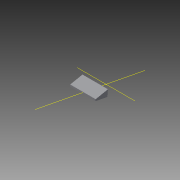
# Autodesk Inventor part: Prow
Saved by Autodesk Inventor 2015 (Build 190159000, 159)
## iProperties
Created: 2016-01-19
Part Number: Prow
Material: Generic
Document SubType Name: Modeling
Designer: sethbattis
Density: 1 g/cm^3
Appearance: Default
Author: sethbattis
Autodesk Inventor part; units mm, degrees
ref_plane "YZ Plane" through (0, 0, 0) normal (1, 0, 0) x (0, 1, 0)
ref_plane "XZ Plane" through (0, 0, 0) normal (0, 1, 0) x (-1, 0, 0)
ref_plane "XY Plane" through (0, 0, 0) normal (0, 0, 1) x (1, 0, 0)
sketch "Robot Front End" plane through (0, 0, 0) normal (1, 0, 0) x (0, 1, 0)
  circle A0 centre (127, -196.85) radius 127
  line L0 (304.8, 0) -> (177.8, 0)
  line L1 (177.8, 0) -> (177.8, 50.8)
  line L2 (209.55, 82.55) -> (273.05, 82.55)
  line L3 (304.8, 50.8) -> (304.8, 0)
  line L4 (0, -1177.7856) -> (0, 1643.8138) projected
  line L5 (-567.69, 0) -> (1050.29, 0) projected
  arc A1 (209.55, 82.55) -> (177.8, 50.8) centre (209.55, 50.8) ccw
  arc A2 (304.8, 50.8) -> (273.05, 82.55) centre (273.05, 50.8) ccw
  line L6 (241.3, 381) -> (0, 381) construction
  circle A3 centre (165.1, -196.85) radius 9.525
  circle A4 centre (241.3, -196.85) radius 25.4
  circle A5 centre (241.3, -196.85) radius 281.427 construction
  circle A6 centre (241.3, -196.85) radius 577.85 construction
  line L7 (165.1, -196.85) -> (241.3, -196.85) construction
  point P0 (0, 0)
  point P1 (177.8, 82.55)
  point P2 (304.8, 82.55)
  dimension "d76" = 254
  dimension "d77" = 127
  dimension "d78" = 82.55
  dimension "d79" = 304.8
  dimension "d80" = 196.85
  dimension "d81" = 31.75
  dimension "d82" = 381
  dimension "d104" = 19.05
  dimension "d105" = 165.1
  dimension "d110" = 50.8
  dimension "d128" = 76.2
  constraints: 12 end point, 6 centre point, 6 tangent, 5 point on line, 4 point on circle, 3 horizontal, 2 coincident, 2 parallel, 2 perpendicular, 1 collinear, 1 equal radius, 1 vertical alignment, 2 other
  measures "d76" diameter of A0
  measures "d77" distance of point (177.8, 82.55) point (304.8, 82.55)
  measures "d78" distance of L0.end point (177.8, 82.55)
  measures "d79" distance between parallel lines of L3 L4
  measures "d80" distance from line of A0.centre L5
  measures "d81" radius of A1
  measures "d82" distance between parallel lines of L5 L6
  measures "d104" diameter of A3
  measures "d105" distance from line of L4 L7.start
  measures "d110" diameter of A4
  measures "d128" distance of L7.start L7.end
sketch "Portcullis" plane through (0, 0, 0) normal (1, 0, 0) x (0, 1, 0)
  line L0 (0, 1071.5852) -> (76.2, 776.4639)
  line L1 (76.2, 776.4639) -> (76.2, 166.8639)
  line L2 (76.2, 166.8639) -> (0, -128.2574)
  line L3 (0, -1177.7856) -> (0, 1643.8138) projected
  line L4 (-567.69, 0) -> (1050.29, 0) projected
  line L5 (76.2, 379.7426) -> (285.0269, 379.7426) construction
  line L6 (203.2, 379.7426) -> (203.2, 475.769)
  line L7 (241.3, 381) -> (0, 381) projected
  circle A0 centre (241.3, -196.85) radius 577.85 construction
  point P0 (0, 0)
  dimension "d83" = 304.8
  dimension "d84" = 609.6
  dimension "d85" = 76.2
  dimension "d86" = 508
  dimension "d87" = 127
  constraints: 10 end point, 4 point on line, 2 vertical, 1 equal length, 1 horizontal, 1 point on circle
  measures "d83" distance of L0.start L0.end
  measures "d84" distance of L0.end L1.end
  measures "d85" distance between parallel lines of L3 L1
  measures "d86" distance from line of L2.end L5
  measures "d87" distance between parallel lines of L1 L6
sketch "Ball Attack" plane through (0, 0, 0) normal (1, 0, 0) x (0, 1, 0)
  line L0 (0, -1177.7856) -> (0, 1643.8138) construction
  circle A0 centre (241.3, -196.85) radius 281.427 construction
  circle A1 centre (241.3, -196.85) radius 577.85 construction
  circle A2 centre (241.3, -196.85) radius 25.4 construction
  circle A3 centre (127, 233.7148) radius 127 construction
  line L1 (112.0448, 53.1385) -> (217.7767, -206.4319)
  line L2 (0, 328.2071) -> (112.0448, 53.1385)
  line L3 (18.1025, 299.0626) -> (94.7574, 110.8758)
  arc A4 (112.0448, 53.1385) -> (0, -52.021) centre (241.3, -196.85) ccw
  line L4 (3.1764, 320.4091) -> (196.7074, 399.2409) construction
  line L5 (98.995, 85.1756) -> (292.526, 164.0074) construction
  line L6 (196.7074, 399.2409) -> (292.526, 164.0074) construction
  line L7 (244.6167, 281.6241) -> (9.3833, 185.8055) construction
  line L8 (0, 328.2071) -> (193.531, 407.0389) construction
  line L9 (111.6779, 54.0392) -> (304.6402, 134.2674) construction
  dimension "d111" = 254
  dimension "d113" = 203.2
  constraints: 18 end point, 8 point on circle, 7 point on line, 5 tangent, 4 perpendicular, 2 centre point, 2 collinear, 1 coincident, 1 midpoint, 1 parallel, 5 other
  measures "d111" diameter of A3
  measures "d113" distance of L3.start L3.end
sketch "Portcullis attack" plane through (0, 0, 0) normal (1, 0, 0) x (0, 1, 0)
  line L0 (203.2, 379.7426) -> (203.2, 475.769) construction
  line L1 (241.3, 381) -> (0, 381) construction
  circle A0 centre (127, -196.85) radius 127 construction
  line L2 (304.8, 50.8) -> (304.8, 0) construction
  arc A1 (304.8, 50.8) -> (273.05, 82.55) centre (273.05, 50.8) ccw construction
  line L3 (209.55, 82.55) -> (273.05, 82.55) construction
  line L4 (202.2679, 382.7157) -> (297.5125, 78.9059)
  line L5 (127, -196.85) -> (127, -196.85) construction
  line L6 (76.2, 776.4639) -> (76.2, 166.8639) construction
  line L7 (76.2, 166.8639) -> (0, -128.2574) construction
  circle A2 centre (165.1, -196.85) radius 9.525 projected
  circle A3 centre (241.3, -196.85) radius 25.4 construction
  circle A4 centre (241.3, -196.85) radius 577.85 construction
  circle A5 centre (241.3, -196.85) radius 281.427 construction
  line L8 (215.9, -196.85) -> (241.3, 381) construction
  arc A6 (228.2571, 84.2746) -> (138.1991, 65.0113) centre (241.3, -196.85) ccw construction
  arc A7 (112.0448, 53.1385) -> (0, -52.021) centre (241.3, -196.85) ccw construction
  line L9 (202.2679, 382.7157) -> (241.3, 381)
  point P0 (0, 0)
  point P1 (0, 381)
  constraints: 8 end point, 4 point on circle, 2 point on line, 1 centre point, 1 coincident, 1 concentric, 1 horizontal alignment, 1 perpendicular, 1 tangent, 1 vertical, 1 vertical alignment, 3 other
sketch "Cheval de Frise" plane through (0, 0, 0) normal (1, 0, 0) x (0, 1, 0)
  line L0 (0, 1240.7281) -> (76.2, 945.6068)
  line L1 (76.2, 945.6068) -> (76.2, 336.0068)
  line L2 (76.2, 336.0068) -> (0, 40.8855)
  line L3 (0, -1177.7856) -> (0, 1643.8138) projected
  line L4 (-567.69, 0) -> (1050.29, 0) projected
  line L5 (171.45, 640.8068) -> (76.2, 640.8068)
  circle A0 centre (171.45, 640.8068) radius 25.4
  line L6 (87.8983, 936.3973) -> (76.2, 931.4537)
  line L7 (76.2, 931.4537) -> (194.8466, 650.694)
  line L8 (313.4933, 369.9343) -> (325.1916, 374.8779)
  line L9 (325.1916, 374.8779) -> (87.8983, 936.3973)
  line L10 (194.8466, 650.694) -> (313.4933, 369.9343)
  circle A1 centre (241.3, -196.85) radius 577.85 construction
  point P0 (0, 0)
  dimension "d92" = 50.8
  dimension "d88" = 304.8
  dimension "d89" = 609.6
  dimension "d90" = 76.2
  dimension "d91" = 95.25
  dimension "d93" = 12.7
  dimension "d94" = 609.6
  constraints: 18 end point, 3 parallel, 3 perpendicular, 3 point on line, 2 equal length, 1 coincident, 1 midpoint, 1 symmetric about line, 1 vertical, 6 other
  measures "d88" distance of L0.start L0.end
  measures "d89" distance of L0.end L1.end
  measures "d90" distance between parallel lines of L3 L1
  measures "d91" distance of L5.start L5.end
  measures "d93" distance of L8.end L8.start
  measures "d94" distance of L8.start L6.end
sketch "Cheval de Frise attack" plane through (0, 0, 0) normal (1, 0, 0) x (0, 1, 0)
  line L0 (0, -1177.7856) -> (0, 1643.8138) construction
  line L1 (325.1916, 374.8779) -> (87.8983, 936.3973) construction
  line L2 (313.4933, 369.9343) -> (325.1916, 374.8779) construction
  line L3 (203.2, 379.7426) -> (297.5125, 78.9059) construction
  line L4 (425.9297, 58.8444) -> (363.6336, 367.9023)
  line L5 (325.1916, 374.8779) -> (363.6336, 367.9023)
  circle A0 centre (241.3, -196.85) radius 577.85 construction
  circle A1 centre (241.3, -196.85) radius 281.427 construction
  circle A2 centre (241.3, -196.85) radius 25.4 construction
  line L6 (0, 328.2071) -> (112.0448, 53.1385) construction
  line L7 (202.2679, 382.7157) -> (241.3, 381) projected
  line L8 (269.1961, 83.191) -> (424.1332, 67.757)
  line L9 (269.1961, 83.191) -> (216.3555, -192.0614)
  line L10 (269.1961, 83.191) -> (325.1916, 374.8779)
  line L11 (241.3, -196.85) -> (294.3571, 79.5303)
  point P0 (0, 0)
  point P1 (0, 381)
  point P2 (200.025, -196.85)
  point P3 (112.0448, 53.1385)
  dimension "d125" = 39.0698
  constraints: 12 end point, 3 equal length, 3 point on circle, 1 collinear, 1 parallel, 1 point on line, 1 tangent, 3 other
  measures "d125" distance of L1.start L4.end
extrude "Extrusion6" add sketch "Cheval de Frise attack" along normal mid plane 622.3
body "Solid5"
